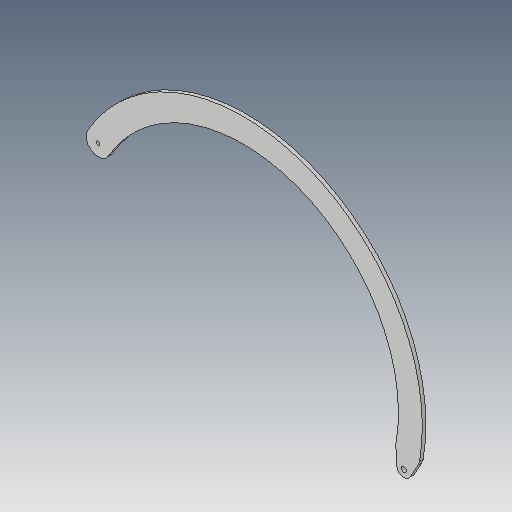
# Autodesk Inventor part: RailWay
Saved by Autodesk Inventor 2019.4 (Build 234330000, 330)
## iProperties
Created: 2019-06-11
Part Number: RailWay
Material: Generic
Document SubType Name: Modeling
Designer: AzLIer
Density: 1 g/cm^3
Appearance: Default
Mass: 24.7622 g
Surface Area: 191.656 cm^2
Volume: 24.7622 cm^3
Author: AzLIer
Autodesk Inventor part; units mm, degrees
ref_plane "YZ Plane" through (0, 0, 0) normal (1, 0, 0) x (0, 1, 0)
ref_plane "XZ Plane" through (0, 0, 0) normal (0, 1, 0) x (-1, 0, 0)
ref_plane "XY Plane" through (0, 0, 0) normal (0, 0, 1) x (1, 0, 0)
sketch "スケッチ1" plane through (0, 0, 0) normal (0, 0, 1) x (1, 0, 0)
  arc A0 (137.8731, -24.3107) -> (-121.2436, 70) centre (0, 0) ccw construction
  arc A1 (147.7212, -26.0472) -> (-129.9038, 75) centre (0, 0) ccw
  arc A2 (128.025, -22.5743) -> (-112.5833, 65) centre (0, 0) ccw
  arc A3 (128.025, -22.5743) -> (147.7212, -26.0472) centre (137.8731, -24.3107) ccw
  arc A4 (-129.9038, 75) -> (-112.5833, 65) centre (-121.2436, 70) ccw
  line L0 (0, 0) -> (0, 140) construction
  circle A5 centre (-121.2436, 70) radius 1.6
  dimension "d0" = 140
  dimension "d1" = 10
  dimension "d4" = 60
  dimension "d5" = 100
  dimension "d6" = 3.2
  constraints: 11 point on circle, 6 centre point, 4 tangent, 2 coincident, 2 end point, 1 vertical
  measures "d0" radius of A0
  measures "d1" radius of A3
  measures "d6" diameter of A5
extrude "押し出し1" add sketch "スケッチ1" along normal blind 3
sketch "スケッチ2" plane through (0, 0, 0) normal (0, 0, -1) x (-1, 0, 0)
  arc A0 (129.9038, 75) -> (-147.7212, -26.0472) centre (0, 0) ccw projected
  arc A1 (-147.7212, -26.0472) -> (-128.025, -22.5743) centre (-137.8731, -24.3107) ccw projected
  arc A2 (112.5833, 65) -> (-128.025, -22.5743) centre (0, 0) ccw projected
  arc A3 (112.5833, 65) -> (129.9038, 75) centre (121.2436, 70) ccw projected
  arc A4 (-137.8731, -24.3107) -> (-134.5766, -38.5892) centre (0, 0) ccw construction
  arc A5 (-139.8324, -41.4835) -> (-128.584, -38.8866) centre (-134.5766, -38.5892) ccw
  line L0 (0, 0) -> (-134.5766, -38.5892) construction
  line L1 (0, 0) -> (-137.8731, -24.3107) construction
  line L2 (-139.8324, -41.4835) -> (-146.6327, -29.1345)
  line L3 (-128.584, -38.8866) -> (-127.8854, -24.8063)
  arc A6 (-147.7212, -26.0472) -> (-128.025, -22.5743) centre (-137.8731, -24.3107) ccw projected
  circle A7 centre (-134.5766, -38.5892) radius 2.1
  dimension "d7" = 6
  dimension "d9" = 6
  dimension "d10" = 4.2
  constraints: 8 end point, 6 point on circle, 4 tangent, 3 centre point, 2 coincident
  measures "d7" angle of L1 L0
  measures "d9" radius of A5
  measures "d10" diameter of A7
extrude "押し出し2" add sketch "スケッチ2" against normal blind 3 contours A1 L3 A5 L2
